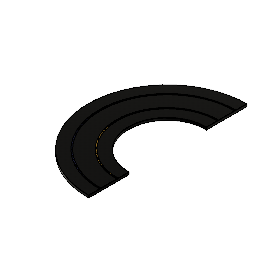
_17-19 (Semicircle).dd4c51f8-2fba-41f0-a670-19c05ef01e43 (Autodesk Fusion 360 design; units mm, degrees)
Autodesk Fusion 360 part; units mm, degrees
sketch "Sketch1" plane through (0, 0, 0) normal (0, 0, 1) x (1, 0, 0)
  line L0 (0, 0) -> (0, -1600.2)
  line L1 (0, -800.1) -> (-812.8, -800.1)
  line L2 (0, -800.1) -> (-1651, -800.1)
  line L3 (0, -1600.2) -> (0, -2438.4)
  line L4 (0, -2438.4) -> (0, -1600.2)
  line L5 (0, 0) -> (0, 838.2)
  circle A0 centre (-12.6008, -800.1) radius 800.1992
  circle A1 centre (-12.6512, -800.1) radius 1638.3488
  dimension "d5" = 838.2
  dimension "d6" = 838.2
  constraint coincident L0.start L5.start
  constraint vertical L0
  constraint horizontal L1
  constraint midpoint L0 L1.start
  constraint perpendicular L0 L2
  constraint perpendicular L2 L3
  constraint parallel L3 L4
  constraint parallel L0 L5
  constraint coincident L0.end A0
  constraint coincident L1.end A0
  constraint coincident L0.start A0
  constraint coincident L3.end A1
  constraint coincident L2.end A1
  constraint coincident L5.end A1
  measures "d5" distance of L3.end L0.end
  measures "d6" distance of L0.start L5.end
extrude "Extrude1" add sketch "Sketch1" along normal blind 50.8 contours L2 L5 A0 A1 | L2 L3 L4 A0 A1
sketch "Sketch2" plane through (0, 0, 50.8) normal (0, 0, 1) x (-1, 0, 0)
  line L0 (0, 0) -> (0, -838.2)
  arc A0 (0, -838.2) -> (0, 2438.4) centre (12.6512, 800.1) ccw
  line L1 (0, 2438.4) -> (0, 1600.2)
  arc A1 (0, 0) -> (0, 1600.2) centre (12.6008, 800.1) ccw
  arc A2 (-3.9498, -250.7939) -> (-3.9498, 1850.9939) centre (12.6008, 800.1) ccw
  arc A3 (-3.6498, -231.7463) -> (-3.6498, 1831.9463) centre (12.6008, 800.1) ccw
  arc A4 (1.9368, -587.3825) -> (1.9368, 2187.5825) centre (12.6512, 800.1) ccw
  arc A5 (1.7897, -606.4319) -> (1.7897, 2206.6319) centre (12.6512, 800.1) ccw
  line L2 (1.9368, 2187.5825) -> (0, 2187.5675)
  line L3 (1.7897, 2206.6319) -> (0, 2206.6181)
  line L4 (1.9368, -587.3825) -> (0, -587.3675)
  line L5 (1.7897, -606.4319) -> (0, -606.4181)
  constraint coincident L1 L2.end
  constraint tangent A4 L2
  constraint coincident L1 L3.end
  constraint tangent A5 L3
  constraint coincident L0 L4.end
  constraint tangent A4 L4
  constraint coincident L0 L5.end
  constraint tangent A5 L5
  constraint parallel L4 L5
extrude "Extrude2" add sketch "Sketch2" along normal blind 0.0279 contours L0 L1 A2 A3
sketch "Sketch3" plane through (0, 0, 50.8) normal (0, 0, 1) x (-1, 0, 0)
  arc A0 (0, -250.8487) -> (0, 1851.0487) centre (12.6008, 800.1) ccw
  line L0 (0, -250.8487) -> (0, -838.2)
  arc A1 (0, -838.2) -> (0, 2438.4) centre (12.6512, 800.1) ccw
  line L1 (0, 2438.4) -> (0, 1851.0487)
  arc A2 (1.9368, -587.3825) -> (1.9368, 2187.5825) centre (12.6512, 800.1) ccw
  arc A3 (1.7897, -606.4319) -> (1.7897, 2206.6319) centre (12.6512, 800.1) ccw
  line L2 (1.7897, -606.4319) -> (0, -606.4181)
  line L3 (1.9368, -587.3825) -> (0, -587.3675)
  line L4 (1.9368, 2187.5825) -> (0, 2187.5825)
  line L5 (1.7897, 2206.6319) -> (0, 2206.6181)
  constraint coincident L0 L2.end
  constraint tangent A3 L2
  constraint coincident L0 L3.end
  constraint tangent A2 L3
  constraint coincident L1 L4.end
  constraint perpendicular L1 L4
  constraint coincident L1 L5.end
  constraint tangent A3 L5
extrude "Extrude3" add sketch "Sketch3" along normal blind 0.0279 contours L0 L1 A2 A3 L2 L3 L4 L5
